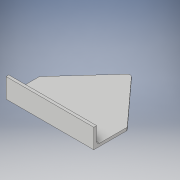
# Autodesk Inventor part: SnowBlowerMotorMount
Saved by Autodesk Inventor 2017.3 (Build 213256000, 256)
## iProperties
Created: 2017-04-27
Part Number: SnowBlowerMotorMount
Material: Generic
Document SubType Name: Modeling
Designer: steele
Density: 1 g/cm^3
Appearance: Default
Author: steele
Autodesk Inventor part; units mm, degrees
ref_plane "YZ Plane" through (0, 0, 0) normal (1, 0, 0) x (0, 1, 0)
ref_plane "XZ Plane" through (0, 0, 0) normal (0, 1, 0) x (-1, 0, 0)
ref_plane "XY Plane" through (0, 0, 0) normal (0, 0, 1) x (1, 0, 0)
sketch "Sketch1" plane through (0, 0, 0) normal (0, 1, 0) x (-1, 0, 0)
  line L0 (0, 0) -> (45.72, 0)
  line L1 (45.72, 0) -> (45.72, -34.798)
  line L2 (45.72, -34.798) -> (0, -85.09)
  line L3 (0, -85.09) -> (0, 0) construction
  line L4 (0, 0) -> (-45.72, 0)
  line L5 (-45.72, 0) -> (-45.72, -34.798)
  line L6 (-45.72, -34.798) -> (0, -85.09)
  dimension "d0" = 45.72
  dimension "d1" = 85.09
  dimension "d2" = 34.798
  constraints: 14 end point, 2 symmetric about line, 1 horizontal, 1 perpendicular, 1 vertical
  measures "d0" distance from line of L0.start L1
  measures "d1" distance of L0.start L2.end
  measures "d2" distance of L0.end L1.end
extrude "Extrusion1" add sketch "Sketch1" along normal blind 2.921
sketch "Sketch3" plane through (0, 2.921, 0) normal (0, 1, 0) x (1, 0, 0)
  line L0 (-45.72, 0) -> (45.72, 0) projected
  line L1 (45.72, 0) -> (45.72, 34.798) projected
  line L2 (-45.72, 0) -> (45.72, 0)
  line L3 (45.72, 0) -> (45.72, 2.921)
  line L4 (45.72, 2.921) -> (-45.72, 2.921)
  line L5 (-45.72, 2.921) -> (-45.72, 0)
  point P0 (0, 0)
  dimension "d5" = 2.921
  constraints: 8 end point, 2 parallel, 1 horizontal, 1 perpendicular, 1 point on line
  measures "d5" distance of L3.end L2.end
extrude "Extrusion2" add sketch "Sketch3" along normal blind 17.399
fillet "Fillet1" radius 3.175 1 edges at (0, 1.4605, -85.09)
fillet "Fillet2" radius 3.175 2 edges at (45.72, 1.4605, -34.798) (-45.72, 1.4605, -34.798)
fillet "Fillet3" radius 3.175 1 edges at (0, 2.921, -2.921)
body "Solid1"
